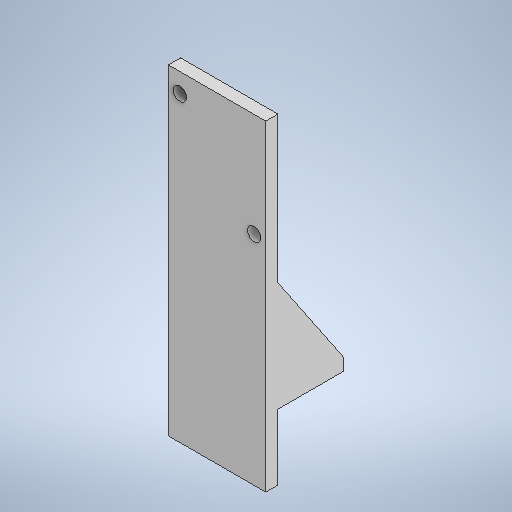
# Autodesk Inventor part: SolenoidMount
Saved by Autodesk Inventor 2025.1 (Build 291241000, 241)
## iProperties
Created: 2025-11-05
Part Number: SolenoidMount
Material: Generic
Document SubType Name: Modeling
Designer: Juxin
Density: 1 g/cm^3
Appearance: Default
Author: Juxin
Autodesk Inventor part; units mm, degrees
ref_plane "YZ Plane" through (0, 0, 0) normal (1, 0, 0) x (0, 1, 0)
ref_plane "XZ Plane" through (0, 0, 0) normal (0, 1, 0) x (-1, 0, 0)
ref_plane "XY Plane" through (0, 0, 0) normal (0, 0, 1) x (1, 0, 0)
sketch "Sketch1" plane through (0, 0, 0) normal (0, 1, 0) x (-1, 0, 0)
  line L0 (0, 0) -> (25.4, 0)
  line L1 (25.4, 0) -> (25.4, -20.32)
  line L2 (25.4, -20.32) -> (0, -20.32)
  line L3 (0, -20.32) -> (0, 0)
  dimension "d0" = 25.4
  dimension "d1" = 20.32
  constraints: 8 end point, 2 parallel, 1 horizontal, 1 perpendicular
  measures "d0" distance of L1.end L2.end
  measures "d1" distance of L0.end L1.end
extrude "Extrusion1" add sketch "Sketch1" along normal blind 3.1623
sketch "Sketch2" plane through (0, 0, 0) normal (0, -1, 0) x (1, 0, 0)
  line L0 (-25.4, 0) -> (0, 0) projected
  line L1 (0, 0) -> (0, -20.32) projected
  line L2 (-25.4, 0) -> (0, 0)
  line L3 (0, 0) -> (0, -3.175)
  line L4 (0, -3.175) -> (-25.4, -3.175)
  line L5 (-25.4, -3.175) -> (-25.4, 0)
  dimension "d4" = 3.175
  constraints: 8 end point, 2 parallel, 1 horizontal, 1 perpendicular, 1 point on line
  measures "d4" distance of L2.end L3.end
extrude "Extrusion2" add sketch "Sketch2" along normal blind 17.145
sketch "Sketch3" plane through (0, 3.1623, 0) normal (0, 1, 0) x (1, 0, 0)
  line L0 (-25.4, 0) -> (0, 0) projected
  line L1 (0, 0) -> (0, 20.32) projected
  line L2 (-25.4, 0) -> (0, 0)
  line L3 (0, 0) -> (0, 3.175)
  line L4 (0, 3.175) -> (-25.4, 3.175)
  line L5 (-25.4, 3.175) -> (-25.4, 0)
  dimension "d7" = 3.175
  constraints: 8 end point, 2 parallel, 1 horizontal, 1 perpendicular, 1 point on line
  measures "d7" distance of L3.end L2.end
extrude "Extrusion3" add sketch "Sketch3" along normal blind 63.5
sketch "Sketch4" plane through (0, 3.1623, -3.175) normal (0, 0, -1) x (-1, 0, 0)
  line L0 (0, 63.5) -> (25.4, 63.5) projected
  line L1 (25.4, 63.5) -> (22.4, 63.5)
  line L2 (22.4, 63.5) -> (22.4, 58.5)
  circle A0 centre (22.4, 58.5) radius 1.75
  line L3 (0, 63.5) -> (3, 63.5)
  line L4 (3, 63.5) -> (3, 36.5)
  circle A1 centre (3, 36.5) radius 1.75
  point P0 (0, -3.1623)
  dimension "d10" = 3
  dimension "d11" = 5
  dimension "d12" = 3.5
  dimension "d13" = 3
  dimension "d14" = 27
  dimension "d15" = 3.5
  constraints: 8 end point, 2 centre point, 2 coincident, 2 perpendicular, 2 point on line
  measures "d10" distance of L0.end L1.end
  measures "d11" distance of L1.end L2.end
  measures "d12" diameter of A0
  measures "d13" distance of L0.start L3.end
  measures "d14" distance of L3.end L4.end
  measures "d15" diameter of A1
extrude "Extrusion4" cut sketch "Sketch4" against normal blind 63.5
sketch "Sketch5" plane through (0, 0, -20.32) normal (1, 0, 0) x (0, 0, -1)
  line L0 (0, 0) -> (0, 3.1623) projected
  line L1 (-17.145, 3.1623) -> (0, 3.1623) projected
  line L2 (0, 3.1623) -> (-17.145, 3.1623)
  line L3 (-17.145, 3.1623) -> (-17.145, 28.5623)
  line L4 (-17.145, 3.1623) -> (-17.145, 66.6623) projected
  line L5 (-17.145, 28.5623) -> (0, 3.1623)
  point P0 (-20.32, 0)
  dimension "d18" = 25.4
  constraints: 6 end point, 1 collinear, 1 point on line
  measures "d18" distance of L1.start L3.end
extrude "Extrusion5" add sketch "Sketch5" against normal blind 3.175
sketch "Sketch6" plane through (-25.4, 0, -20.32) normal (-1, 0, 0) x (0, 0, 1)
  line L0 (17.145, 28.5623) -> (0, 3.1623) projected
  line L1 (0, 3.1623) -> (17.145, 3.1623) projected
  line L2 (0, 3.1623) -> (17.145, 3.1623)
  line L3 (17.145, 3.1623) -> (17.145, 28.5508)
  line L4 (17.145, 28.5508) -> (0, 3.1623)
  point P0 (20.32, 0)
  constraints: 6 end point, 1 horizontal, 1 perpendicular
extrude "Extrusion6" add sketch "Sketch6" against normal blind 3.175
body "Solid1"
